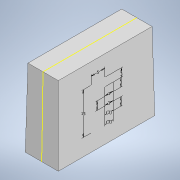
# Autodesk Inventor part: Gembok
Saved by Autodesk Inventor 2021 (Build 250183000, 183)
## iProperties
Created: 2022-03-10
Part Number: Gembok
Material: Generic
Document SubType Name: Modeling
Designer: User
Density: 1 g/cm^3
Appearance: Default
Author: User
Autodesk Inventor part; units mm, degrees
ref_plane "YZ Plane" through (0, 0, 0) normal (1, 0, 0) x (0, 1, 0)
ref_plane "XZ Plane" through (0, 0, 0) normal (0, 1, 0) x (-1, 0, 0)
ref_plane "XY Plane" through (0, 0, 0) normal (0, 0, 1) x (1, 0, 0)
sketch "Sketch1" plane through (0, 0, 0) normal (0, 1, 0) x (-1, 0, 0)
  line L0 (5.9069, 17.9943) -> (-6.0931, 17.9943)
  line L1 (-6.0931, 17.9943) -> (-6.0931, -17.0057)
  line L2 (-6.0931, -17.0057) -> (5.9069, -17.0057)
  line L3 (5.9069, -17.0057) -> (5.9069, 17.9943)
  point P0 (0, 0)
  dimension "d0" = 12
  dimension "d1" = 35
  constraints: 8 end point, 2 parallel, 1 horizontal, 1 perpendicular
  measures "d0" distance of L2.end L1.end
  measures "d1" distance of L1.end L0.end
extrude "Extrusion1" add sketch "Sketch1" along normal blind 28 draft -1
sketch "Sketch3" plane through (0, 0, 0) normal (1, 0, 0) x (0, 1, 0)
  line L0 (28, -16.5169) -> (0, -17.0057) projected
  line L1 (0, -17.0057) -> (0, 17.9943) projected
  line L2 (0, 17.9943) -> (28, 17.5056) projected
  line L3 (28, 17.5056) -> (28, -16.5169) projected
  line L4 (0, 0) -> (15, 0)
  line L5 (15, 0) -> (15, -5)
  line L6 (15, -5) -> (12, -5)
  line L7 (12, -5) -> (12, -8)
  line L8 (12, -8) -> (9, -8)
  line L9 (9, -8) -> (9, -5)
  line L10 (9, -5) -> (6, -5)
  line L11 (6, -5) -> (6, -8)
  line L12 (6, -8) -> (3, -8)
  line L13 (3, -8) -> (3, -5)
  line L14 (3, -5) -> (0, -5)
  line L15 (0, -17.0057) -> (0, 17.9943) projected
  line L16 (0, 0) -> (0, -5)
  dimension "d9" = 15
  dimension "d10" = 5
  dimension "d11" = 3
  dimension "d12" = 3
  dimension "d13" = 3
  dimension "d14" = 3
  dimension "d15" = 3
  dimension "d16" = 3
  dimension "d17" = 3
  dimension "d18" = 3
  constraints: 24 end point, 7 point on line, 5 perpendicular, 1 horizontal
  measures "d9" distance of L4.start L4.end
  measures "d10" distance of L4.end L5.end
  measures "d11" distance of L5.end L6.end
  measures "d12" distance of L6.end L7.end
  measures "d13" distance of L7.end L8.end
  measures "d14" distance of L8.end L9.end
  measures "d15" distance of L9.end L10.end
  measures "d16" distance of L10.end L11.end
  measures "d17" distance of L11.end L12.end
  measures "d18" distance of L12.end L13.end
body "Solid1"
